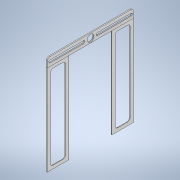
# Autodesk Inventor part: Part On Monitor
Saved by Autodesk Inventor 2020.2 (Build 242310000, 310)
## iProperties
Created: 2020-05-07
Part Number: Part On Monitor
Material: Generic
Document SubType Name: Modeling
Designer: Amaan Khalid
Density: 1 g/cm^3
Appearance: Default
Author: Amaan Khalid
Autodesk Inventor part; units mm, degrees
ref_plane "YZ Plane" through (0, 0, 0) normal (1, 0, 0) x (0, 1, 0)
ref_plane "XZ Plane" through (0, 0, 0) normal (0, 1, 0) x (-1, 0, 0)
ref_plane "XY Plane" through (0, 0, 0) normal (0, 0, 1) x (1, 0, 0)
sketch "Sketch1" plane through (0, 0, 0) normal (1, 0, 0) x (0, 1, 0)
  line L0 (7.6752, 16.382) -> (7.6752, -31.243)
  line L1 (7.6752, 16.382) -> (7.6752, 64.007)
  line L2 (-2.4848, 16.382) -> (-2.4848, 64.007)
  line L3 (0.6902, 67.182) -> (4.5002, 67.182)
  line L4 (-2.4848, 16.382) -> (-2.4848, -31.243)
  line L5 (0.6902, -34.418) -> (4.5002, -34.418)
  arc A0 (7.6752, 64.007) -> (4.5002, 67.182) centre (4.5002, 64.007) ccw
  arc A1 (4.5002, -34.418) -> (7.6752, -31.243) centre (4.5002, -31.243) ccw
  line L6 (-2.4848, 64.007) -> (-2.4848, 67.182)
  line L7 (-2.4848, 67.182) -> (0.6902, 67.182)
  line L8 (-2.4848, -31.243) -> (-2.4848, -34.418)
  line L9 (0.6902, -34.418) -> (-2.4848, -34.418)
  circle A2 centre (2.5952, 16.382) radius 4
  point P0 (0, 0)
  point P1 (7.6752, -34.418)
  point P2 (7.6752, 67.182)
  dimension "d1" = 50.8
  dimension "d2" = 50.8
  dimension "d3" = 3.175
  dimension "d101" = 8
  constraints: 20 end point, 8 point on line, 4 point on circle, 4 tangent, 4 vertical, 3 centre point, 3 perpendicular, 1 equal radius, 1 horizontal
  measures "d1" distance of L0.start point (7.675, -34.418)
  measures "d2" distance of L0.start point (7.675, 67.182)
  measures "d3" radius of A0
  measures "d101" diameter of A2
extrude "Extrusion1" add sketch "Sketch1" along normal blind 1.27 contours L0 A1 L5 L9 L8 L4 L2 L6 L7 L3 A0 L1 | A2
sketch "Sketch4" plane through (0, -2.4848, 16.382) normal (0, -1, 0) x (1, 0, 0)
  line L0 (1.27, 50.8) -> (1.27, -50.8) projected
  line L1 (1.27, 0) -> (1.27, 47.625) projected
  line L2 (0.9525, 50.8) -> (0.9525, 25.4)
  line L3 (0.9525, 50.8) -> (0.3175, 50.8)
  line L4 (0.3175, 50.8) -> (0.3175, 25.4)
  line L5 (0.3175, 25.4) -> (0.9525, 25.4)
  line L6 (0, -50.8) -> (1.27, -50.8) projected
  line L7 (0.9525, -50.8) -> (0.9525, -25.4)
  line L8 (0.9525, -25.4) -> (0.3175, -25.4)
  line L9 (0.3175, -25.4) -> (0.3175, -50.8)
  line L10 (0.9525, -50.8) -> (0.3175, -50.8)
  point P0 (0, -16.382)
  dimension "d27" = 25.4
  dimension "d28" = 0.635
  dimension "d29" = 25.4
  dimension "d31" = 25.4
  dimension "d32" = 0.635
  constraints: 16 end point, 5 perpendicular, 2 point on line, 1 vertical
  measures "d27" distance of L2.start L2.end
  measures "d28" distance of L2.start L3.end
  measures "d29" distance of L3.end L4.end
  measures "d31" distance of L7.start L7.end
  measures "d32" distance of L7.end L8.end
extrude "Extrusion3" add sketch "Sketch4" along normal blind 106.68
sketch "Sketch5" plane through (0.9525, -2.4848, 67.182) normal (1, 0, 0) x (0, 0, -1)
  line L0 (0, 6.985) -> (0, 0) projected
  line L1 (0, 0) -> (0, -106.68) projected
  line L2 (25.4, 0) -> (25.4, -106.68) projected
  line L3 (0, 0) -> (101.6, 0) projected
  line L4 (6.985, -3.81) -> (18.415, -3.81)
  line L5 (21.59, -6.985) -> (21.59, -99.695)
  line L6 (18.415, -102.87) -> (6.985, -102.87)
  line L7 (3.81, -99.695) -> (3.81, -6.985)
  line L8 (25.4, -106.68) -> (0, -106.68) projected
  arc A0 (6.985, -3.81) -> (3.81, -6.985) centre (6.985, -6.985) ccw
  arc A1 (21.59, -6.985) -> (18.415, -3.81) centre (18.415, -6.985) ccw
  arc A2 (3.81, -99.695) -> (6.985, -102.87) centre (6.985, -99.695) ccw
  arc A3 (18.415, -102.87) -> (21.59, -99.695) centre (18.415, -99.695) ccw
  line L9 (83.185, -3.81) -> (94.615, -3.81)
  line L10 (97.79, -6.985) -> (97.79, -99.695)
  line L11 (94.615, -102.87) -> (83.185, -102.87)
  line L12 (80.01, -99.695) -> (80.01, -6.985)
  line L13 (101.6, 0) -> (101.6, -106.68) projected
  line L14 (50.8, 0) -> (101.6, 0) projected
  line L15 (76.2, 0) -> (76.2, -106.68) projected
  line L16 (101.6, -106.68) -> (76.2, -106.68) projected
  arc A4 (83.185, -3.81) -> (80.01, -6.985) centre (83.185, -6.985) ccw
  arc A5 (97.79, -6.985) -> (94.615, -3.81) centre (94.615, -6.985) ccw
  arc A6 (80.01, -99.695) -> (83.185, -102.87) centre (83.185, -99.695) ccw
  arc A7 (94.615, -102.87) -> (97.79, -99.695) centre (94.615, -99.695) ccw
  point P0 (67.182, 2.4848)
  dimension "d67" = 3.81
  dimension "d68" = 3.81
  dimension "d69" = 3.81
  dimension "d70" = 3.81
  dimension "d71" = 3.175
  dimension "d72" = 3.81
  dimension "d73" = 3.81
  dimension "d74" = 3.81
  dimension "d75" = 3.81
  dimension "d76" = 3.175
  constraints: 16 end point, 16 point on circle, 16 tangent, 8 centre point, 6 equal radius, 4 parallel, 2 horizontal, 2 perpendicular
  measures "d67" distance between parallel lines of L6 L8
  measures "d68" distance between parallel lines of L3 L4
  measures "d69" distance between parallel lines of L2 L5
  measures "d70" distance between parallel lines of L1 L7
  measures "d71" radius of A0
  measures "d72" distance between parallel lines of L13 L10
  measures "d73" distance between parallel lines of L14 L9
  measures "d74" distance between parallel lines of L15 L12
  measures "d75" distance between parallel lines of L16 L11
  measures "d76" radius of A4
extrude "Extrusion5" cut sketch "Sketch5" against normal through all contours L4 A1 L5 A3 L6 A2 L7 A0 | L9 A5 L10 A7 L11 A6 L12 A4
sketch "Sketch6" plane through (1.27, 0, 0) normal (1, 0, 0) x (0, 0, -1)
  line L0 (-67.182, -2.4848) -> (34.418, -2.4848) projected
  line L1 (-16.382, 7.6752) -> (-64.007, 7.6752) projected
  line L2 (-41.782, -2.4848) -> (-67.182, -2.4848) projected
  arc A0 (-64.007, 4.1192) -> (-64.007, 1.0712) centre (-64.007, 2.5952) ccw
  arc A1 (-16.382, 7.6752) -> (-16.382, -2.4848) centre (-16.382, 2.5952) ccw projected
  arc A2 (-24.637, 1.0712) -> (-24.637, 4.1192) centre (-24.637, 2.5952) ccw
  line L3 (-64.007, 4.1192) -> (-24.637, 4.1192)
  line L4 (-64.007, 1.0712) -> (-24.637, 1.0712)
  point P0 (0, 0)
  dimension "d90" = 3.048
  constraints: 4 end point, 4 point on circle, 2 centre point, 1 horizontal, 1 tangent
  measures "d90" diameter of A2
extrude "Extrusion6" cut sketch "Sketch6" against normal through all
sketch "Sketch7" plane through (1.27, 0, 0) normal (1, 0, 0) x (0, 0, -1)
  arc A0 (-16.382, -2.4848) -> (-16.382, 7.6752) centre (-16.382, 2.5952) ccw projected
  arc A1 (-8.127, 4.1192) -> (-8.127, 1.0712) centre (-8.127, 2.5952) ccw
  arc A2 (31.2702, 1.0712) -> (31.2702, 4.1192) centre (31.2702, 2.5952) ccw
  line L0 (31.2702, 4.1192) -> (-8.127, 4.1192)
  line L1 (-8.127, 1.0712) -> (31.2702, 1.0712)
  point P0 (0, 0)
  dimension "d96" = 3.048
  dimension "d98" = 3.048
  constraints: 4 end point, 4 point on circle, 2 centre point, 1 horizontal, 1 tangent
  measures "d96" diameter of A1
  measures "d98" diameter of A2
extrude "Extrusion7" cut sketch "Sketch7" against normal through all
sketch "Sketch8" plane through (1.27, 0, 0) normal (1, 0, 0) x (0, 0, -1)
  arc A0 (-24.637, 1.0712) -> (-24.637, 4.1192) centre (-24.637, 2.5952) ccw projected
  circle A1 centre (-16.382, 2.5952) radius 4
  point P0 (0, 0)
  dimension "d103" = 8
  constraints: 1 centre point
  measures "d103" diameter of A1
extrude "Extrusion8" cut sketch "Sketch8" against normal through all
body "Solid1"
